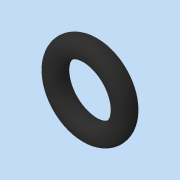
# Autodesk Inventor part: wiringTubingORings
Saved by Autodesk Inventor 2017 (Build 210142000, 142)
## iProperties
Created: 2017-04-25
Part Number: wiringTubingORings
Material: Rubber, Nitrile
Document SubType Name: Modeling
Designer: Derek Wider
Mass: 0.0584862 g
Surface Area: 1.09648 cm^2
Volume: 0.0487385 cm^3
Density: 1.2 g/cm^3
Appearance: Rubber - Black
Author: Derek Wider
Autodesk Inventor part; units mm, degrees
ref_plane "YZ Plane" through (0, 0, 0) normal (1, 0, 0) x (0, 1, 0)
ref_plane "XZ Plane" through (0, 0, 0) normal (0, 1, 0) x (-1, 0, 0)
ref_plane "XY Plane" through (0, 0, 0) normal (0, 0, 1) x (1, 0, 0)
sketch "Sketch1" plane through (0, 0, 0) normal (1, 0, 0) x (0, 1, 0)
  circle A0 centre (3.1242, 0) radius 0.889
  line L0 (0, 0) -> (0, 1.6314)
  dimension "d0" = 1.778
  dimension "d1" = 3.1242
  constraints: 2 end point, 1 centre point, 1 vertical
  measures "d0" diameter of A0
  measures "d1" distance of L0.start A0.centre
revolve "Revolution1" add sketch "Sketch1" angle 360 about axis through (0, 0, 0) along (0, 0, 1)
body "Solid1"
